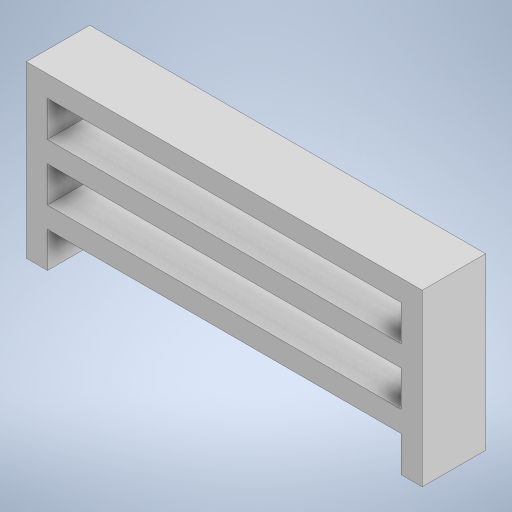
# Autodesk Inventor part: Large Shelves
Saved by Autodesk Inventor 2023 (Build 270158000, 158)
## iProperties
Created: 2022-11-15
Part Number: Large Shelves
Material: Generic
Document SubType Name: Modeling
Designer: Team 4026
Density: 1 g/cm^3
Appearance: Default
Author: Team 4026
Autodesk Inventor part; units mm, degrees
ref_plane "YZ Plane" through (0, 0, 0) normal (1, 0, 0) x (0, 1, 0)
ref_plane "XZ Plane" through (0, 0, 0) normal (0, 1, 0) x (-1, 0, 0)
ref_plane "XY Plane" through (0, 0, 0) normal (0, 0, 1) x (1, 0, 0)
sketch "Sketch2" plane through (0, 0, 0) normal (0, 1, 0) x (-1, 0, 0)
  line L0 (0, 0) -> (-3810, 0)
  line L1 (-3810, 0) -> (-3810, -609.6)
  line L2 (-3810, -609.6) -> (0, -609.6)
  line L3 (0, -609.6) -> (0, 0)
  dimension "d2" = 609.6
  dimension "d3" = 3810
  constraints: 8 end point, 2 parallel, 1 horizontal, 1 perpendicular
  measures "d2" distance of L2.end L0.start
  measures "d3" distance of L0.start L0.end
extrude "Extrusion1" add sketch "Sketch2" along normal blind 546.1
shell "Shell1" thickness 203.2 removed faces 3 at (1270, 364.0667, 0) at (2540, 364.0667, -609.6) at (2540, 0, -203.2)
pattern_linear "Rectangular Pattern1" count 3 spacing 546.1 along (0, 1, 0)
equation "\"d4\" = shelfheight"
equation "\"d8\" = shelfheight"
equation "\"totalheight\" = 1638.3"
equation "\"shelfheight\" = 546.1"
body "Solid1"
